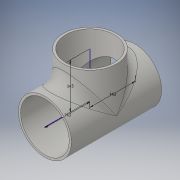
# Autodesk Inventor part: 6in tee sch40
Saved by Autodesk Inventor 2016 (Build 200138000, 138)
## iProperties
Created: 2016-08-28
Part Number: 6in tee sch40
Material: Generic
Document SubType Name: Modeling
Designer: Luiz Henrique
Density: 1 g/cm^3
Appearance: Default
Author: Luiz Henrique
Autodesk Inventor part; units mm, degrees
ref_plane "YZ Plane" through (0, 0, 0) normal (1, 0, 0) x (0, 1, 0)
ref_plane "XZ Plane" through (0, 0, 0) normal (0, 1, 0) x (-1, 0, 0)
ref_plane "XY Plane" through (0, 0, 0) normal (0, 0, 1) x (1, 0, 0)
sketch "Sketch6" plane through (0, 0, 0) normal (1, 0, 0) x (0, 1, 0)
  line L0 (0, 0) -> (0, 143)
  line L1 (0, 0) -> (0, -143)
  line L2 (0, 0) -> (143, 0)
  dimension "d4" = 143
  dimension "d5" = 143
  dimension "d6" = 143
  constraints: 6 end point, 2 vertical, 1 horizontal
  measures "d4" distance of L0.start L0.end
  measures "d5" distance of L0.start L1.end
  measures "d6" distance of L0.start L2.end
sketch "Sketch7" plane through (0, 0, 0) normal (0, 0, 1) x (1, 0, 0)
  circle A0 centre (0, 0) radius 84
  circle A1 centre (0, 0) radius 76.89
  dimension "d7" = 168
  dimension "d8" = 7.11
  constraints: 2 centre point, 1 coincident
  measures "d7" diameter of A0
  measures "d8" radial gap between concentric circles of A0 A1
sketch "Sketch8" plane through (0, 0, 0) normal (0, 1, 0) x (-1, 0, 0)
  circle A0 centre (0, 0) radius 84
  circle A1 centre (0, 0) radius 76.89
  dimension "d9" = 168
  dimension "d10" = 7.11
  constraints: 2 centre point, 1 coincident
  measures "d9" diameter of A0
  measures "d10" radial gap between concentric circles of A0 A1
extrude "Extrusion2" add sketch "Sketch7" along normal mid plane 286
extrude "Extrusion3" add sketch "Sketch8" along normal blind 143
sketch "Sketch9" plane through (0, 0, -143) normal (0, 0, -1) x (-1, 0, 0)
  circle A0 centre (0, 0) radius 77.0342
  constraints: 1 centre point, 1 coincident
extrude "Extrusion4" cut sketch "Sketch9" against normal blind 300
sketch "Sketch10" plane through (0, 143, 0) normal (0, 1, 0) x (1, 0, 0)
  circle A0 centre (0, 0) radius 76.89
  constraints: 1 centre point, 1 coincident
extrude "Extrusion5" cut sketch "Sketch10" against normal blind 143
fillet "Fillet1" radius 40 2 edges at (0, 84, 84) (0, 84, -84)
body "Solid2"
